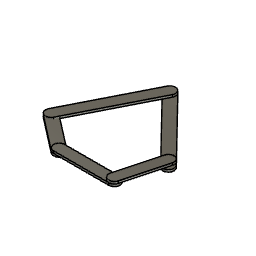
five bar mechanism (Autodesk Fusion 360 design; units mm, degrees)
Autodesk Fusion 360 part; units mm, degrees
sketch "Sketch1" plane through (0, 0, 0) normal (0, 0, 1) x (1, 0, 0)
  line L0 (0, -5) -> (50, -5)
  arc A0 (50, -5) -> (50, 5) centre (50, 0) ccw
  line L1 (50, 5) -> (0, 5)
  arc A1 (0, 5) -> (0, -5) centre (0, 0) ccw
  line L2 (0, 0) -> (50, 0) construction
  line L3 (0, -20) -> (40, -20)
  arc A2 (40, -20) -> (40, -10) centre (40, -15) ccw
  line L4 (40, -10) -> (0, -10)
  arc A3 (0, -10) -> (0, -20) centre (0, -15) ccw
  line L5 (0, -15) -> (40, -15) construction
  line L6 (0, -35) -> (40, -35)
  arc A4 (40, -35) -> (40, -25) centre (40, -30) ccw
  line L7 (40, -25) -> (0, -25)
  arc A5 (0, -25) -> (0, -35) centre (0, -30) ccw
  line L8 (0, -30) -> (40, -30) construction
  line L9 (0, -50) -> (80, -50)
  arc A6 (80, -50) -> (80, -40) centre (80, -45) ccw
  line L10 (80, -40) -> (0, -40)
  arc A7 (0, -40) -> (0, -50) centre (0, -45) ccw
  line L11 (0, -45) -> (80, -45) construction
  line L12 (0, -65) -> (80, -65)
  arc A8 (80, -65) -> (80, -55) centre (80, -60) ccw
  line L13 (80, -55) -> (0, -55)
  arc A9 (0, -55) -> (0, -65) centre (0, -60) ccw
  line L14 (0, -60) -> (80, -60) construction
  dimension "d75" = 50
  dimension "d76" = 5
  dimension "d77" = 80
  dimension "d78" = 40
  constraint tangent L0 A0
  constraint tangent A0 L1
  constraint parallel L0 L1
  constraint tangent L1 A1
  constraint tangent L0 A1
  constraint horizontal L2
  constraint coincident A1.centre L2.start
  constraint tangent L3 A2
  constraint tangent A2 L4
  constraint parallel L3 L4
  constraint tangent L4 A3
  constraint tangent L3 A3
  constraint horizontal L5
  constraint tangent L6 A4
  constraint tangent A4 L7
  constraint parallel L6 L7
  constraint tangent L7 A5
  constraint tangent L6 A5
  constraint horizontal L8
  constraint tangent L9 A6
  constraint tangent A6 L10
  constraint parallel L9 L10
  constraint tangent L10 A7
  constraint tangent L9 A7
  constraint horizontal L11
  constraint tangent L12 A8
  constraint tangent A8 L13
  constraint parallel L12 L13
  constraint tangent L13 A9
  constraint tangent L12 A9
  constraint horizontal L14
  measures "d75" distance of A0.end L1.end
  measures "d76" radius of A0
  measures "d77" distance of L12.start L12.end
  measures "d78" distance of L6.start L6.end
extrude "Extrude1" add sketch "Sketch1" along normal blind 2 makes body 1 at (26.6667, -31.6667, 0) makes body 2 at (26.6667, -16.6667, 0) makes body 3 at (53.3333, -46.6667, 0) makes body 4 at (33.3333, -1.6667, 0) makes body 5 at (53.3333, -61.6667, 0) in component "Component"
copy_body "Body->Comp1" bodies 1 removing the originals makes body 6 in component "Component'"
copy_body "Body->Comp2" bodies 2 removing the originals makes body 7 in component "Component''"
copy_body "Body->Comp3" bodies 3 removing the originals makes body 8 in component "Component'''"
copy_body "Body->Comp4" bodies 4 removing the originals makes body 9 in component "Component''''"
copy_body "Body->Comp5" bodies 5 removing the originals makes body 10 in component "Component'''''"
component "Component" placed x (1, 0, 0) y (0, 1, 0) z (0, 0, 1) at (0, 0, 0)
component "Component'" placed x (0.910245, -0.41407, 0) y (-0.41407, -0.910245, 0) z (0, 0, -1) at (-48.8319, -10.7445, 0) in component "Component"
component "Component''" placed x (0.98753, -0.157431, 0) y (-0.157431, -0.98753, 0) z (0, 0, -1) at (8.1373, -8.5157, 4) in component "Component"
component "Component'''" placed x (-0.08925, 0.996009, 0) y (0.996009, 0.08925, 0) z (0, 0, -1) at (15.5507, -59.1017, 2) in component "Component"
component "Component''''" placed x (1, 0, 0) y (0, 1, 0) z (0, 0, 1) at (0, 0, 0) in component "Component"
component "Component'''''" placed x (-0.497107, -0.867689, 0) y (0.867689, -0.497107, 0) z (0, 0, 1) at (62.5602, -23.5292, -2) in component "Component"
